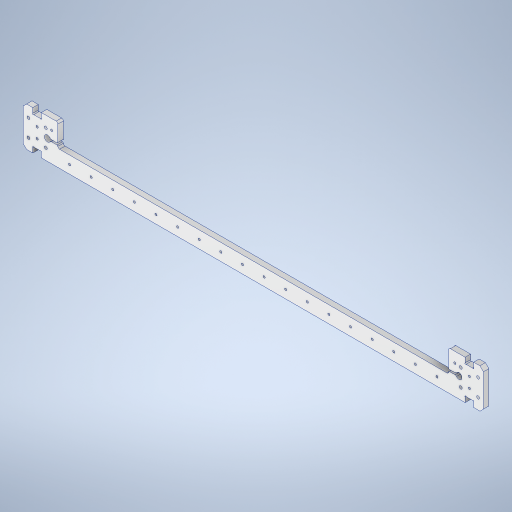
# Autodesk Inventor part: R3 Gantry Bar
Saved by Autodesk Inventor 2024 (Build 280153000, 153)
## iProperties
Created: 2024-08-05
Part Number: R3 Gantry Bar
Material: Aluminum 6061
Document SubType Name: Modeling
Designer: Ishaan
Density: 2.7 g/cm^3
Appearance: Aluminum - Flat
Author: Ishaan
Autodesk Inventor part; units mm, degrees
ref_plane "YZ Plane" through (0, 0, 0) normal (1, 0, 0) x (0, 1, 0)
sketch "Sketch1" plane through (0, 0, 0) normal (0, 0, 1) x (1, 0, 0)
  line L0 (-236.5, -22.7) -> (-263.5, -22.7)
  line L1 (-263.5, -22.7) -> (-263.5, 22.7)
  line L2 (-263.5, 22.7) -> (-236.5, 22.7)
  line L3 (-236.5, 22.7) -> (-236.5, -22.7)
  line L4 (-236.5, -22.7) -> (-263.5, 22.7) construction
  line L5 (-263.5, -22.7) -> (-236.5, 22.7) construction
  line L6 (236.5, -22.7) -> (263.5, -22.7)
  line L7 (263.5, -22.7) -> (263.5, 22.7)
  line L8 (263.5, 22.7) -> (236.5, 22.7)
  line L9 (236.5, 22.7) -> (236.5, -22.7)
  line L10 (236.5, -22.7) -> (263.5, 22.7) construction
  line L11 (263.5, -22.7) -> (236.5, 22.7) construction
  line L12 (-236.5, 2.7) -> (-236.5, 22.7)
  line L13 (236.5, 22.7) -> (236.5, 18.0393)
  line L14 (250, -22.7) -> (-250, -22.7)
  line L15 (-250, -22.7) -> (-250, -3.5)
  line L16 (-250, -3.5) -> (250, -3.5)
  line L17 (250, -3.5) -> (250, -22.7)
  line L18 (250, -22.7) -> (-250, -3.5) construction
  line L19 (-250, -22.7) -> (250, -3.5) construction
  point P0 (0, 0)
  point P1 (0, 0)
  point P2 (-250, 0)
  point P3 (0, -13.1)
  point P4 (-250, 0)
  point P5 (250, 0)
  point P6 (236.5, -3.5)
  point P7 (-236.5, -3.5)
  point P8 (-236.5, -22.7)
  point P9 (236.5, -22.7)
  dimension "d1" = 27
  dimension "d2" = 45.4
  dimension "d97" = 500
  dimension "d98" = 19.2
  constraints: 40 end point, 9 parallel, 5 midpoint, 4 collinear, 3 horizontal, 3 perpendicular, 2 point on line, 1 coincident, 1 horizontal alignment, 1 vertical alignment
  measures "d1" distance of L1.end L2.end
  measures "d2" distance of L0.end L1.end
  measures "d97" distance of L15.end L16.end
  measures "d98" distance between parallel lines of L14 L16
extrude "Extrusion1" add sketch "Sketch1" against normal blind 6.35
sketch "Sketch2" plane through (0, 0, -6.35) normal (0, 0, -1) x (1, 0, 0)
  line L0 (-240, -10) -> (-260, -10) construction
  line L1 (-260, -10) -> (-260, 10) construction
  line L2 (-260, 10) -> (-240, 10) construction
  line L3 (-240, 10) -> (-240, -10) construction
  line L4 (-240, -10) -> (-260, 10) construction
  line L5 (-260, -10) -> (-240, 10) construction
  line L6 (260, -10) -> (240, -10) construction
  line L7 (240, -10) -> (240, 10) construction
  line L8 (240, 10) -> (260, 10) construction
  line L9 (260, 10) -> (260, -10) construction
  line L10 (260, -10) -> (240, 10) construction
  line L11 (240, -10) -> (260, 10) construction
  point P0 (0, 0)
  point P1 (-250, 0)
  point P2 (250, 0)
  point P3 (-250, 0)
  point P4 (250, 0)
  dimension "d8" = 20
  dimension "d9" = 20
  dimension "d10" = 20
  dimension "d11" = 20
  constraints: 24 end point, 10 coincident, 4 midpoint, 4 parallel, 2 horizontal, 2 perpendicular
  measures "d8" distance of L1.end L2.end
  measures "d9" distance of L0.end L1.end
  measures "d10" distance of L7.end L8.end
  measures "d11" distance of L6.end L7.end
hole "Hole1" at (-260, -10, -6.35) at (-240, -10, -6.35) at (-240, 10, -6.35) at (-260, 10, -6.35) at (240, -10, -6.35) at (260, -10, -6.35) at (260, 10, -6.35) at (240, 10, -6.35) direction (0, 0, 1) diameter 3.3 end through all
sketch "Sketch3" plane through (0, 0, -6.35) normal (0, 0, -1) x (1, 0, 0)
  circle A0 centre (240, -10) radius 1.65 projected
  circle A1 centre (260, -10) radius 1.65 projected
  circle A2 centre (260, 10) radius 1.65 projected
  circle A3 centre (240, 10) radius 1.65 projected
  circle A4 centre (-260, -10) radius 1.65 projected
  circle A5 centre (-240, -10) radius 1.65 projected
  circle A6 centre (-240, 10) radius 1.65 projected
  circle A7 centre (-260, 10) radius 1.65 projected
  line L0 (-263.5, 22.7) -> (-263.5, -22.7) projected
  line L1 (-236.5, -22.7) -> (-236.5, 3.5) projected
  line L2 (236.5, 3.5) -> (236.5, -22.7) projected
  line L3 (263.5, -22.7) -> (263.5, 22.7) projected
  line L4 (-263.5, -22.7) -> (-236.5, -22.7) projected
  line L5 (240, 10) -> (260, -10) construction
  line L6 (266.2, 22.7) -> (233.8, 22.7)
  line L7 (233.8, 22.7) -> (233.8, -22.7)
  line L8 (233.8, -22.7) -> (266.2, -22.7)
  line L9 (266.2, -22.7) -> (266.2, 22.7)
  line L10 (266.2, 22.7) -> (233.8, -22.7) construction
  line L11 (233.8, 22.7) -> (266.2, -22.7) construction
  line L12 (263.5, 22.7) -> (-263.5, 22.7) projected
  line L13 (236.5, -22.7) -> (263.5, -22.7) projected
  line L14 (-236.5, 3.5) -> (236.5, 3.5) projected
  line L15 (266.2, -16.2) -> (233.8, -16.2)
  line L16 (233.8, -16.2) -> (233.8, 16.2)
  line L17 (233.8, 16.2) -> (266.2, 16.2)
  line L18 (266.2, 16.2) -> (266.2, -16.2)
  line L19 (266.2, -16.2) -> (233.8, 16.2) construction
  line L20 (233.8, -16.2) -> (266.2, 16.2) construction
  line L21 (-266.2, 22.7) -> (-233.8, 22.7)
  line L22 (-233.8, 22.7) -> (-233.8, -22.7)
  line L23 (-233.8, -22.7) -> (-266.2, -22.7)
  line L24 (-266.2, -22.7) -> (-266.2, 22.7)
  line L25 (-266.2, 22.7) -> (-233.8, -22.7) construction
  line L26 (-233.8, 22.7) -> (-266.2, -22.7) construction
  line L27 (-266.2, 16.2) -> (-233.8, 16.2)
  line L28 (-233.8, 16.2) -> (-233.8, -16.2)
  line L29 (-233.8, -16.2) -> (-266.2, -16.2)
  line L30 (-266.2, -16.2) -> (-266.2, 16.2)
  line L31 (-266.2, 16.2) -> (-233.8, -16.2) construction
  line L32 (-233.8, 16.2) -> (-266.2, -16.2) construction
  point P0 (0, 0)
  point P1 (250, 0)
  point P2 (263.5, -22.7)
  point P3 (263.5, 22.7)
  point P4 (211.5, -16.2)
  point P5 (233.8, 3.5)
  point P6 (233.8, 22.7)
  point P7 (-250, 0)
  point P8 (250, -16.2)
  point P9 (-263.5, -16.2)
  point P10 (-263.5, 16.2)
  point P11 (-266.2, 16.2)
  point P12 (-236.5, -22.7)
  point P13 (-233.8, 3.5)
  point P14 (263.5, -16.2)
  point P15 (266.2, -16.2)
  point P16 (266.2, 16.2)
  point P17 (263.5, 16.2)
  point P18 (228.8, 22.7)
  point P19 (228.8, -22.7)
  point P20 (221.2, -22.7)
  point P21 (263.5, 22.7)
  point P22 (263.5, -22.7)
  point P23 (-233.8, 22.7)
  point P24 (-221.2, -22.7)
  point P25 (-228.8, -22.7)
  point P26 (-228.8, 22.7)
  point P27 (233.8, -16.2)
  point P28 (-263.5, 22.7)
  point P29 (-263.5, -22.7)
  dimension "d100" = 32.4
  dimension "d102" = 6.2
  dimension "d103" = 6.2
  constraints: 50 end point, 10 midpoint, 8 parallel, 4 perpendicular, 3 collinear, 3 horizontal, 3 point on line
  measures "d100" distance between parallel lines of L17 L15
  measures "d102" distance from line of L17 A2.centre
  measures "d103" distance from line of L18 A2.centre
extrude "Extrusion8" add sketch "Sketch3" against normal up to surface (6.35 mm away) contours L0 L27 L24 L21 | L0 L29 L24 L27 | L0 L23 L24 L29 | L29 L22 L23 L1 | L1 L14 L22 L29 | L6 L9 L17 L3 | L14 L2 L15 L7 | L17 L9 L15 L3 | L15 L2 L8 L7 | L15 L9 L8 L3
sketch "Sketch4" plane through (0, 0, -6.35) normal (0, 0, -1) x (1, 0, 0)
  circle A0 centre (240, -10) radius 1.65 construction
  circle A1 centre (260, -10) radius 1.65 construction
  circle A2 centre (260, 10) radius 1.65 construction
  circle A3 centre (240, 10) radius 1.65 construction
  circle A4 centre (-260, -10) radius 1.65 construction
  circle A5 centre (-240, -10) radius 1.65 construction
  circle A6 centre (-240, 10) radius 1.65 construction
  circle A7 centre (-260, 10) radius 1.65 construction
  line L0 (-233.8, -22.7) -> (-233.8, 3.5) construction
  line L1 (-233.8, 3.5) -> (233.8, 3.5) construction
  line L2 (233.8, 3.5) -> (233.8, -22.7) construction
  line L3 (233.8, -22.7) -> (266.2, -22.7) construction
  line L4 (266.2, -22.7) -> (266.2, 22.7) construction
  line L5 (-266.2, 22.7) -> (-266.2, -22.7) construction
  line L6 (233.8, 3.5) -> (-233.8, 3.5) construction
  line L7 (-233.8, 3.5) -> (-233.8, 22.7) construction
  line L8 (-233.8, 22.7) -> (233.8, 22.7) construction
  line L9 (233.8, 22.7) -> (233.8, 3.5) construction
  line L10 (-266.2, -22.7) -> (-233.8, -22.7) projected
  line L11 (266.2, 22.7) -> (-266.2, 22.7) projected
  line L12 (-212.5, 13.1) -> (212.5, 13.1) construction
  point P0 (187.5, 13.1)
  point P1 (162.5, 13.1)
  point P2 (137.5, 13.1)
  point P3 (112.5, 13.1)
  point P4 (87.5, 13.1)
  point P5 (62.5, 13.1)
  point P6 (37.5, 13.1)
  point P7 (12.5, 13.1)
  point P8 (-12.5, 13.1)
  point P9 (-37.5, 13.1)
  point P10 (-62.5, 13.1)
  point P11 (-87.5, 13.1)
  point P12 (-112.5, 13.1)
  point P13 (-137.5, 13.1)
  point P14 (-162.5, 13.1)
  point P15 (0, 3.5)
  point P16 (-233.8, 13.1)
  point P17 (-187.5, 13.1)
  point P18 (0, 13.1)
  point P19 (0, 3.5)
  dimension "d108" = 25
  constraints: 10 end point, 4 midpoint, 3 equal length, 2 horizontal, 1 collinear, 1 perpendicular, 1 point on line, 1 vertical alignment, 17 other
  measures "d108" distance of L12.end point (187.5, 13.1)
hole "Hole2" at (-162.5, -13.1, -6.35) at (-137.5, -13.1, -6.35) at (-112.5, -13.1, -6.35) at (-87.5, -13.1, -6.35) at (-62.5, -13.1, -6.35) at (-37.5, -13.1, -6.35) at (-12.5, -13.1, -6.35) at (12.5, -13.1, -6.35) at (37.5, -13.1, -6.35) at (62.5, -13.1, -6.35) at (87.5, -13.1, -6.35) at (112.5, -13.1, -6.35) at (137.5, -13.1, -6.35) at (162.5, -13.1, -6.35) at (187.5, -13.1, -6.35) at (212.5, -13.1, -6.35) at (-187.5, -13.1, -6.35) at (-212.5, -13.1, -6.35) direction (0, 0, 1) diameter 2.459 end through all thread size "M3x0.5" class "6H" standard "ANSI Metric M Profile"
sketch "Sketch5" plane through (0, 0, -6.35) normal (0, 0, -1) x (1, 0, 0)
  circle A0 centre (240, -10) radius 1.65 projected
  circle A1 centre (260, -10) radius 1.65 projected
  circle A2 centre (260, 10) radius 1.65 projected
  circle A3 centre (240, 10) radius 1.65 projected
  circle A4 centre (-260, -10) radius 1.65 projected
  circle A5 centre (-240, -10) radius 1.65 projected
  circle A6 centre (-240, 10) radius 1.65 projected
  circle A7 centre (-260, 10) radius 1.65 projected
  line L0 (226, -0.4) -> (238, -0.4) construction
  line L1 (226, -1.4) -> (238, -1.4)
  line L2 (238, 0.6) -> (226, 0.6)
  arc A8 (226, 0.6) -> (226, -1.4) centre (226, -0.4) ccw
  arc A9 (238, -1.4) -> (238, 0.6) centre (238, -0.4) ccw
  circle A10 centre (238, -0.4) radius 3.5
  circle A11 centre (212.5, 13.1) radius 1.2295 projected
  circle A12 centre (212.5, 13.1) radius 1.2295 projected
  circle A13 centre (187.5, 13.1) radius 1.2295 projected
  circle A14 centre (162.5, 13.1) radius 1.2295 projected
  circle A15 centre (137.5, 13.1) radius 1.2295 projected
  circle A16 centre (112.5, 13.1) radius 1.2295 projected
  circle A17 centre (87.5, 13.1) radius 1.2295 projected
  circle A18 centre (62.5, 13.1) radius 1.2295 projected
  circle A19 centre (37.5, 13.1) radius 1.2295 projected
  circle A20 centre (12.5, 13.1) radius 1.2295 projected
  circle A21 centre (-12.5, 13.1) radius 1.2295 projected
  circle A22 centre (-37.5, 13.1) radius 1.2295 projected
  circle A23 centre (-62.5, 13.1) radius 1.2295 projected
  circle A24 centre (-87.5, 13.1) radius 1.2295 projected
  circle A25 centre (-112.5, 13.1) radius 1.2295 projected
  circle A26 centre (-137.5, 13.1) radius 1.2295 projected
  circle A27 centre (-162.5, 13.1) radius 1.2295 projected
  circle A28 centre (240, -10) radius 1.65 projected
  circle A29 centre (260, -10) radius 1.65 projected
  circle A30 centre (260, 10) radius 1.65 projected
  circle A31 centre (240, 10) radius 1.65 projected
  circle A32 centre (-260, -10) radius 1.65 projected
  circle A33 centre (-240, -10) radius 1.65 projected
  circle A34 centre (-240, 10) radius 1.65 projected
  circle A35 centre (-260, 10) radius 1.65 projected
  line L3 (-233.8, -22.7) -> (-233.8, 3.5) projected
  line L4 (-233.8, 3.5) -> (233.8, 3.5) projected
  line L5 (233.8, 3.5) -> (233.8, -22.7) projected
  line L6 (233.8, -22.7) -> (266.2, -22.7) projected
  line L7 (266.2, -22.7) -> (266.2, 22.7) projected
  line L8 (-266.2, 22.7) -> (-266.2, -22.7) projected
  line L9 (233.8, -22.7) -> (226, -22.7)
  line L10 (226, -22.7) -> (226, 3.5)
  line L11 (226, 3.5) -> (233.8, 3.5)
  line L12 (233.8, 3.5) -> (233.8, -22.7)
  line L13 (-266.2, -22.7) -> (-233.8, -22.7) projected
  line L14 (266.2, 22.7) -> (-266.2, 22.7) projected
  point P0 (0, 0)
  point P1 (232, -0.4)
  point P2 (234.6459, 0.6)
  point P3 (234.6459, -1.4)
  point P4 (250, 0)
  dimension "d46" = 2
  dimension "d48" = 7
  dimension "d49" = 12
  dimension "d113" = 13.5
  dimension "d114" = 12
  constraints: 16 end point, 4 point on circle, 4 tangent, 3 centre point, 3 parallel, 2 horizontal, 2 point on line, 1 coincident, 1 midpoint, 1 perpendicular
  measures "d46" distance between parallel lines of L1 L2
  measures "d48" diameter of A10
  measures "d49" distance of L0.start L0.end
  measures "d113" distance from line of L0 A11.centre
  measures "d114" horizontal distance of L0.end point (250, 0)
extrude "Extrusion9" add sketch "Sketch5" against normal up to surface (6.35 mm away) contours L10 L2 L5 L1 | L1 L5 L9 L10 | L10 L4 L5 L2
extrude "Extrusion4" cut sketch "Sketch5" against normal through all contours L10 L2 L5 L1 | A8 L10 | L5 L2 A10 L1 | A10 L2 A9 L1 | L1 A9 L2 A10
fillet "Fillet1" radius 2 2 edges at (234.6459, -0.6, -3.175) (234.6459, 1.4, -3.175)
mirror "Mirror1" about plane through (0, 0, 0) normal (1, 0, 0) of "Extrusion4", "Fillet1", "Extrusion9"
sketch "Sketch7" plane through (0, 0, -6.35) normal (0, 0, -1) x (1, 0, 0)
  arc A0 (-233.3902, -1.4) -> (-235.0665, -2.3091) centre (-233.3902, -3.4) ccw projected
  arc A1 (-235.0665, 1.5091) -> (-235.0665, -2.3091) centre (-238, -0.4) ccw projected
  arc A2 (-235.0665, 1.5091) -> (-233.3902, 0.6) centre (-233.3902, 2.6) ccw projected
  line L0 (-233.3902, 0.6) -> (-226, 0.6) projected
  line L1 (226, 0.6) -> (233.3902, 0.6) projected
  arc A3 (233.3902, 0.6) -> (235.0665, 1.5091) centre (233.3902, 2.6) ccw projected
  arc A4 (235.0665, -2.3091) -> (235.0665, 1.5091) centre (238, -0.4) ccw projected
  arc A5 (235.0665, -2.3091) -> (233.3902, -1.4) centre (233.3902, -3.4) ccw projected
  line L2 (233.3902, -1.4) -> (226, -1.4) projected
  line L3 (-226, -1.4) -> (-233.3902, -1.4) projected
  circle A6 centre (240, -10) radius 1.65 projected
  circle A7 centre (260, -10) radius 1.65 projected
  circle A8 centre (260, 10) radius 1.65 projected
  circle A9 centre (240, 10) radius 1.65 projected
  circle A10 centre (-260, -10) radius 1.65 projected
  circle A11 centre (-240, -10) radius 1.65 projected
  circle A12 centre (-240, 10) radius 1.65 projected
  circle A13 centre (-260, 10) radius 1.65 projected
  line L4 (-226, 3.5) -> (-226, 0.6) projected
  line L5 (-226, 3.5) -> (226, 3.5) projected
  line L6 (226, 3.5) -> (226, 0.6) projected
  line L7 (226, -1.4) -> (226, -22.7) projected
  line L8 (226, -22.7) -> (266.2, -22.7) projected
  line L9 (266.2, -22.7) -> (266.2, 22.7) projected
  line L10 (-266.2, 22.7) -> (-266.2, -22.7) projected
  line L11 (-226, -1.4) -> (-226, -22.7) projected
  line L12 (245.125, 22.7) -> (254.875, 22.7)
  line L13 (254.875, 22.7) -> (254.875, -22.7)
  line L14 (254.875, -22.7) -> (245.125, -22.7)
  line L15 (245.125, -22.7) -> (245.125, 22.7)
  line L16 (245.125, 22.7) -> (254.875, -22.7) construction
  line L17 (254.875, 22.7) -> (245.125, -22.7) construction
  line L18 (245.125, 16.2) -> (254.875, 16.2)
  line L19 (254.875, 16.2) -> (254.875, -16.2)
  line L20 (254.875, -16.2) -> (245.125, -16.2)
  line L21 (245.125, -16.2) -> (245.125, 16.2)
  line L22 (245.125, 16.2) -> (254.875, -16.2) construction
  line L23 (254.875, 16.2) -> (245.125, -16.2) construction
  line L24 (266.2, 22.7) -> (-266.2, 22.7) projected
  line L25 (-266.2, -22.7) -> (-226, -22.7) projected
  point P0 (0, 0)
  point P1 (250, 0)
  point P2 (250, 16.2)
  point P3 (245.125, -22.7)
  point P4 (254.875, -22.7)
  point P5 (254.875, 16.2)
  point P6 (220.125, 1.5762)
  point P7 (220.125, -1.5762)
  point P8 (245.125, 22.7)
  point P9 (254.875, 22.7)
  dimension "d117" = 9.75
  dimension "d118" = 32.4
  constraints: 24 end point, 5 midpoint, 4 parallel, 2 horizontal, 2 perpendicular, 1 collinear, 1 point on line
  measures "d117" distance of L13.end L14.end
  measures "d118" distance from line of point (250, 16.2) L20
extrude "Extrusion5" cut sketch "Sketch7" against normal up to surface (6.35 mm away) contours L12 L13 L18 L15 | L20 L13 L8 L15
mirror "Mirror2" about plane through (0, 0, 0) normal (1, 0, 0) of "Extrusion5"
sketch "Sketch8" plane through (0, 0, -6.35) normal (0, 0, -1) x (1, 0, 0)
  line L0 (266.2, -22.7) -> (266.2, 22.7) projected
  line L1 (226, 0.6) -> (233.3902, 0.6) projected
  arc A0 (233.3902, 0.6) -> (235.0665, 1.5091) centre (233.3902, 2.6) ccw projected
  arc A1 (235.0665, -2.3091) -> (235.0665, 1.5091) centre (238, -0.4) ccw projected
  arc A2 (235.0665, -2.3091) -> (233.3902, -1.4) centre (233.3902, -3.4) ccw projected
  line L2 (233.3902, -1.4) -> (226, -1.4) projected
  line L3 (-226, -1.4) -> (-233.3902, -1.4) projected
  arc A3 (-233.3902, -1.4) -> (-235.0665, -2.3091) centre (-233.3902, -3.4) ccw projected
  arc A4 (-235.0665, 1.5091) -> (-235.0665, -2.3091) centre (-238, -0.4) ccw projected
  arc A5 (-235.0665, 1.5091) -> (-233.3902, 0.6) centre (-233.3902, 2.6) ccw projected
  line L4 (-233.3902, 0.6) -> (-226, 0.6) projected
  circle A6 centre (-260, 10) radius 1.65 projected
  circle A7 centre (-240, 10) radius 1.65 projected
  circle A8 centre (-240, -10) radius 1.65 projected
  circle A9 centre (-260, -10) radius 1.65 projected
  circle A10 centre (240, 10) radius 1.65 projected
  circle A11 centre (260, 10) radius 1.65 projected
  circle A12 centre (260, -10) radius 1.65 projected
  circle A13 centre (240, -10) radius 1.65 projected
  circle A14 centre (245.525, -16.6) radius 0.75
  line L5 (-254.875, 16.2) -> (-254.875, 22.7) projected
  line L6 (-254.875, 22.7) -> (-266.2, 22.7) projected
  line L7 (-266.2, 22.7) -> (-266.2, -22.7) projected
  line L8 (-266.2, -22.7) -> (-254.875, -22.7) projected
  line L9 (-245.125, -16.2) -> (-245.125, -22.7) projected
  line L10 (-245.125, -22.7) -> (-226, -22.7) projected
  line L11 (-226, -1.4) -> (-226, -22.7) projected
  line L12 (-226, 3.5) -> (-226, 0.6) projected
  line L13 (-226, 3.5) -> (226, 3.5) projected
  line L14 (226, 3.5) -> (226, 0.6) projected
  line L15 (226, -1.4) -> (226, -22.7) projected
  line L16 (226, -22.7) -> (245.125, -22.7) projected
  line L17 (245.125, -22.7) -> (245.125, -16.2) projected
  line L18 (254.875, -16.2) -> (254.875, -22.7) projected
  line L19 (254.875, -22.7) -> (266.2, -22.7) projected
  line L20 (266.2, 22.7) -> (254.875, 22.7) projected
  line L21 (245.125, 22.7) -> (-245.125, 22.7) projected
  line L22 (245.125, -16.2) -> (254.875, -16.2) projected
  line L23 (254.875, 22.7) -> (254.875, 16.2) projected
  line L24 (254.875, 16.2) -> (245.125, 16.2) projected
  line L25 (245.125, 16.2) -> (245.125, 22.7) projected
  line L26 (-245.125, 22.7) -> (-245.125, 16.2) projected
  line L27 (-245.125, 16.2) -> (-254.875, 16.2) projected
  line L28 (-254.875, -22.7) -> (-254.875, -16.2) projected
  line L29 (-254.875, -16.2) -> (-245.125, -16.2) projected
  point P0 (0, 0)
  dimension "d77" = 1.5
  dimension "d141" = 0.4
  dimension "d142" = 0.4
  constraints: 1 centre point
  measures "d77" diameter of A14
  measures "d141" distance from line of L22 A14.centre
  measures "d142" distance from line of A14.centre L17
extrude "Extrusion7" cut sketch "Sketch8" against normal through all contours L22 L17 A14 | A14 L17 L22 | A6 | A7 | A8 | A9 | A10 | A11 | A12 | A13
ref_plane "Work Plane1" through (250, 16.2, -6.35) normal (1, 0, 0) x (0, 0, -1)
mirror "Mirror3" about plane through (250, 16.2, -6.35) normal (1, 0, 0) of "Extrusion7"
ref_plane "Work Plane2" through (246.1594, 0, 0) normal (0, 1, 0) x (1, 0, 0)
mirror "Mirror4" about plane through (246.1594, 0, 0) normal (0, 1, 0) of "Extrusion7", "Mirror3"
mirror "Mirror5" about plane through (0, 0, 0) normal (1, 0, 0) of "Extrusion7", "Mirror3", "Mirror4"
sketch "Sketch9" plane through (0, 0, 0) normal (0, 0, 1) x (1, 0, 0)
  circle A0 centre (212.5, -13.1) radius 1.2295 projected
  point P0 (0, 0)
  point P1 (233.2, 10.9)
  dimension "d119" = 24
  dimension "d120" = 20.7
  measures "d119" vertical distance of point (233.2, 10.9) A0.centre
  measures "d120" horizontal distance of point (233.2, 10.9) A0.centre
hole "Hole4" at (233.2, 10.9, 0) direction (0, 0, -1) diameter 2.459 end through all thread size "M3x0.5" class "6H" standard "ANSI Metric M Profile"
mirror "Mirror6" about plane through (0, 0, 0) normal (1, 0, 0) of "Hole4"
chamfer "Chamfer1" distance 4 angle 45 4 edges at (-266.2, -22.7, -3.175) (-266.2, 22.7, -3.175) (266.2, -22.7, -3.175) (266.2, 22.7, -3.175)
fillet "Fillet9" radius 2 4 edges at (226, 22.7, -3.175) (226, -3.5, -3.175) (-226, -3.5, -3.175) (-226, 22.7, -3.175)
fillet "Fillet10" radius 1 4 edges at (-226, -0.6, -3.175) (-226, 1.4, -3.175) (226, -0.6, -3.175) (226, 1.4, -3.175)
sketch "Sketch10" plane through (0, 0, 0) normal (0, 0, 1) x (1, 0, 0)
  line L0 (-250, 6) -> (-250, -6) construction
  point P0 (0, 0)
  point P1 (-250, 0)
  point P2 (-250, 0)
  dimension "d133" = 12
  constraints: 2 end point, 1 coincident, 1 midpoint, 1 vertical
  measures "d133" distance of L0.start L0.end
hole "Hole5" at (-250, 6, 0) at (-250, -6, 0) direction (0, 0, -1) diameter 2.459 end through all thread size "M3x0.5" class "6H" standard "ANSI Metric M Profile"
mirror "Mirror7" about plane through (0, 0, 0) normal (1, 0, 0) of "Hole5"
equation "\"d103\" = d102"
body "Solid1"
